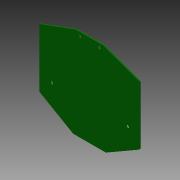
# Autodesk Inventor part: Middle Plate Veroboard
Saved by Autodesk Inventor 2015 (Build 190159000, 159)
## iProperties
Created: 2015-11-27
Part Number: Middle Plate Veroboard
Material: ABS Plastic
Document SubType Name: Modeling
Designer: James
Density: 1.06 g/cm^3
Appearance: Smooth - White
Author: James
Autodesk Inventor part; units mm, degrees
ref_plane "YZ Plane" through (0, 0, 0) normal (1, 0, 0) x (0, 1, 0)
ref_plane "XZ Plane" through (0, 0, 0) normal (0, 1, 0) x (-1, 0, 0)
ref_plane "XY Plane" through (0, 0, 0) normal (0, 0, 1) x (1, 0, 0)
sketch "Sketch1" plane through (0, 0, 0) normal (0, 1, 0) x (-1, 0, 0)
  circle A0 centre (-19.6128, 0) radius 1.6
  circle A1 centre (0, 0) radius 1.6
  circle A2 centre (-48.5529, -55.6025) radius 1.6
  circle A3 centre (28.9401, -55.6025) radius 1.6
  line L0 (-23.9442, 3.8794) -> (-59.8846, -9.2018)
  line L1 (-61.2006, -11.0812) -> (-61.2006, -68.5261)
  line L2 (-60.2006, -70.2582) -> (-27.0236, -89.4129)
  line L3 (4.3314, 3.8794) -> (40.2717, -9.2018)
  line L4 (41.5877, -11.0812) -> (41.5877, -68.5261)
  line L5 (40.5877, -70.2582) -> (7.4108, -89.4129)
  line L6 (-26.0236, -89.6808) -> (6.4108, -89.6808)
  line L7 (-23.2602, 4) -> (3.6473, 4)
  arc A4 (-23.2602, 4) -> (-23.9442, 3.8794) centre (-23.2602, 2) ccw
  arc A5 (4.3314, 3.8794) -> (3.6473, 4) centre (3.6473, 2) ccw
  arc A6 (41.5877, -11.0812) -> (40.2717, -9.2018) centre (39.5877, -11.0812) ccw
  arc A7 (40.5877, -70.2582) -> (41.5877, -68.5261) centre (39.5877, -68.5261) ccw
  arc A8 (6.4108, -89.6808) -> (7.4108, -89.4129) centre (6.4108, -87.6808) ccw
  arc A9 (-27.0236, -89.4129) -> (-26.0236, -89.6808) centre (-26.0236, -87.6808) ccw
  arc A10 (-61.2006, -68.5261) -> (-60.2006, -70.2582) centre (-59.2006, -68.5261) ccw
  arc A11 (-59.8846, -9.2018) -> (-61.2006, -11.0812) centre (-59.2006, -11.0812) ccw
  constraints: 16 end point, 16 point on circle, 12 centre point
extrude "Extrusion1" add sketch "Sketch1" along normal blind 1
body "Solid1"
